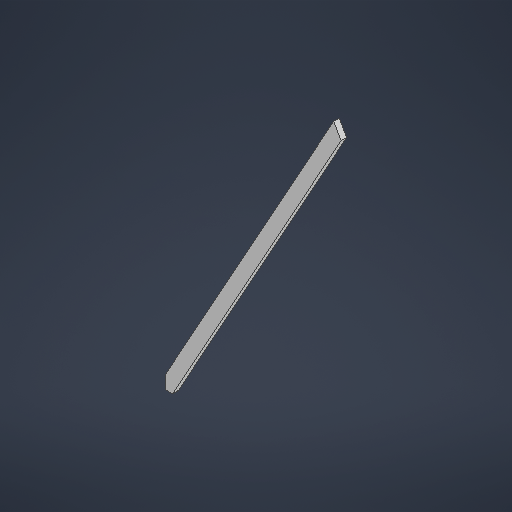
# Autodesk Inventor part: S_2x4x97.048
Saved by Autodesk Inventor 2026 (Build 300175000, 175)
## iProperties
Created: 2025-09-04
Part Number: S_2x4x97.048
Material: Generic
Document SubType Name: Modeling
Designer: trott
Density: 1 g/cm^3
Appearance: Default
Author: trott
Autodesk Inventor part; units mm, degrees
ref_plane "YZ Plane" through (0, 0, 0) normal (1, 0, 0) x (0, 1, 0)
ref_plane "XZ Plane" through (0, 0, 0) normal (0, 1, 0) x (-1, 0, 0)
ref_plane "XY Plane" through (0, 0, 0) normal (0, 0, 1) x (1, 0, 0)
sketch "Sketch1" plane through (0, 0, 0) normal (0, 0, 1) x (1, 0, 0)
  line L0 (-609.6, -2197.1) -> (609.6, -2197.1)
  line L1 (609.6, -2197.1) -> (609.6, 2197.1)
  line L2 (609.6, 2197.1) -> (-609.6, 2197.1)
  line L3 (-609.6, 2197.1) -> (-609.6, -2197.1)
  line L4 (-609.6, -2197.1) -> (609.6, 2197.1) construction
  line L5 (609.6, -2197.1) -> (-609.6, 2197.1) construction
  line L6 (-609.6, 0) -> (609.6, 0)
  line L7 (609.6, 0) -> (-609.6, -2197.1)
  line L8 (-570.7331, -2218.6678) -> (-648.4669, -2175.5322)
  line L9 (648.4669, -21.5678) -> (570.7331, 21.5678)
  line L10 (570.7331, 21.5678) -> (-648.4669, -2175.5322)
  line L11 (-570.7331, -2218.6678) -> (648.4669, -21.5678)
  line L12 (570.7331, 21.5678) -> (609.6, 91.6091)
  line L13 (-609.6, 2197.1) -> (609.6, -2197.1) construction
  line L14 (609.6, 0) -> (-609.6, 2197.1)
  line L15 (-570.7331, 2218.6678) -> (-648.4669, 2175.5322)
  line L16 (648.4669, 21.5678) -> (570.7331, -21.5678)
  line L17 (570.7331, -21.5678) -> (-648.4669, 2175.5322)
  line L18 (-570.7331, 2218.6678) -> (648.4669, 21.5678)
  line L19 (570.7331, -21.5678) -> (609.6, -91.6091)
  point P0 (0, 0)
  point P1 (609.6, 91.6091)
  point P2 (-558.7649, 2197.1)
  point P3 (-609.6, 2105.4909)
  point P4 (609.6, -91.6091)
  point P5 (609.6, -91.6091)
  point P6 (558.7649, 0)
  point P7 (-609.6, -2105.4909)
  point P8 (-558.7649, -2197.1)
  dimension "d0" = 1219.2
  dimension "d1" = 4394.2
  dimension "d3" = 88.9
  dimension "d4" = 88.9
  constraints: 40 end point, 6 midpoint, 5 symmetric about line, 3 perpendicular, 3 point on line, 2 parallel, 1 horizontal
  measures "d0" distance of L2.end L1.end
  measures "d1" distance of L0.end L1.end
  measures "d3" distance of L8.start L8.end
  measures "d4" distance of L9.start L9.end
extrude "Extrusion1" add sketch "Sketch1" along normal blind 38.1 contours L7 L19 L11 L0 | L3 L10 L17 L19 L7
body "Solid1"
